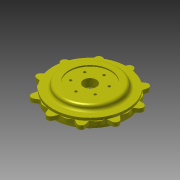
# Autodesk Inventor part: 基准图-主动轮
Saved by Autodesk Inventor 2015 (Build 190159000, 159)
## iProperties
Created: 2017-05-02
Part Number: 基准图-主动轮
Material: 常规
Document SubType Name: Modeling
Designer: Administrator
Density: 1 g/cm^3
Appearance: 黄色
Author: Administrator
Autodesk Inventor part; units mm, degrees
ref_plane "YZ Plane" through (0, 0, 0) normal (1, 0, 0) x (0, 1, 0)
ref_plane "XZ Plane" through (0, 0, 0) normal (0, 1, 0) x (-1, 0, 0)
ref_plane "XY Plane" through (0, 0, 0) normal (0, 0, 1) x (1, 0, 0)
sketch "草图1" plane through (0, 0, 0) normal (0, 0, 1) x (1, 0, 0)
  circle A0 centre (0, 0) radius 141.3842
  line L0 (-50, 166.3842) -> (50, 166.3842)
  line L1 (50, 166.3842) -> (50, 141.3842)
  line L2 (50, 141.3842) -> (-50, 141.3842)
  line L3 (-50, 141.3842) -> (-50, 166.3842)
  line L4 (0, 0) -> (34.0656, 0)
  line L5 (0, 0) -> (0, 40.0691)
  line L6 (-10, 166.3842) -> (-20, 141.3842)
  line L7 (10, 166.3842) -> (20, 141.3842)
  arc A1 (18.8622, 166.3842) -> (13.2913, 158.1558) centre (18.8622, 160.3842) ccw
  arc A2 (18.4913, 145.1558) -> (24.0622, 141.3842) centre (24.0622, 147.3842) ccw
  arc A3 (-13.2913, 158.1558) -> (-18.8622, 166.3842) centre (-18.8622, 160.3842) ccw
  arc A4 (-24.0622, 141.3842) -> (-18.4913, 145.1558) centre (-24.0622, 147.3842) ccw
  circle A5 centre (0, 0) radius 143.3355
  arc A6 (13.2913, 158.1558) -> (-13.2913, 158.1558) centre (0, 152.8393) ccw
  line L8 (-138.249, 105.2184) -> (-57.3473, 163.9969)
  line L9 (-57.3473, 163.9969) -> (-42.6527, 143.7715)
  line L10 (-42.6527, 143.7715) -> (-123.5544, 84.9929)
  line L11 (-123.5544, 84.9929) -> (-138.249, 105.2184)
  line L12 (-173.6916, 3.8627) -> (-142.7899, 98.9684)
  line L13 (-142.7899, 98.9684) -> (-119.0135, 91.2429)
  line L14 (-119.0135, 91.2429) -> (-149.9152, -3.8627)
  line L15 (-149.9152, -3.8627) -> (-173.6916, 3.8627)
  line L16 (-142.7899, -98.9684) -> (-173.6916, -3.8627)
  line L17 (-173.6916, -3.8627) -> (-149.9152, 3.8627)
  line L18 (-149.9152, 3.8627) -> (-119.0135, -91.2429)
  line L19 (-119.0135, -91.2429) -> (-142.7899, -98.9684)
  line L20 (-57.3473, -163.9969) -> (-138.249, -105.2184)
  line L21 (-138.249, -105.2184) -> (-123.5544, -84.9929)
  line L22 (-123.5544, -84.9929) -> (-42.6527, -143.7715)
  line L23 (-42.6527, -143.7715) -> (-57.3473, -163.9969)
  line L24 (50, -166.3842) -> (-50, -166.3842)
  line L25 (-50, -166.3842) -> (-50, -141.3842)
  line L26 (-50, -141.3842) -> (50, -141.3842)
  line L27 (50, -141.3842) -> (50, -166.3842)
  line L28 (-105.8883, 128.7298) -> (-99.2839, 102.6265)
  line L29 (-89.708, 140.4855) -> (-66.9232, 126.1379)
  arc A7 (-70.3607, 128.3025) -> (-63.6368, 128.5256) centre (-67.1635, 133.3797) ccw
  arc A8 (-102.5703, 100.2388) -> (-100.2803, 106.5646) centre (-106.097, 105.0929) ccw
  arc A9 (-82.2087, 135.7632) -> (-103.7146, 120.1383) centre (-89.8367, 123.6496) ccw
  line L30 (-161.3309, 41.905) -> (-140.6447, 24.669)
  line L31 (-155.1506, 60.9261) -> (-128.284, 62.7112)
  arc A10 (-132.3373, 62.4419) -> (-127.0287, 66.5746) centre (-132.7351, 68.4287) ccw
  arc A11 (-141.9, 20.8056) -> (-143.7655, 27.2693) centre (-147.6063, 22.6597) ccw
  arc A12 (-146.3079, 61.5137) -> (-154.5224, 36.232) centre (-145.3588, 47.2299) ccw
  line L32 (-155.1506, -60.9261) -> (-128.284, -62.7112)
  line L33 (-161.3309, -41.905) -> (-140.6447, -24.669)
  arc A13 (-143.7655, -27.2693) -> (-141.9, -20.8056) centre (-147.6063, -22.6597) ccw
  arc A14 (-127.0287, -66.5746) -> (-132.3373, -62.4419) centre (-132.7351, -68.4287) ccw
  arc A15 (-154.5224, -36.232) -> (-146.3079, -61.5137) centre (-145.3588, -47.2299) ccw
  line L34 (-89.708, -140.4855) -> (-66.9232, -126.1379)
  line L35 (-105.8883, -128.7298) -> (-99.2839, -102.6265)
  arc A16 (-100.2803, -106.5646) -> (-102.5703, -100.2388) centre (-106.097, -105.0929) ccw
  arc A17 (-63.6368, -128.5256) -> (-70.3607, -128.3025) centre (-67.1635, -133.3797) ccw
  arc A18 (-103.7146, -120.1383) -> (-82.2087, -135.7632) centre (-89.8367, -123.6496) ccw
  line L36 (10, -166.3842) -> (20, -141.3842)
  line L37 (-10, -166.3842) -> (-20, -141.3842)
  arc A19 (-18.4913, -145.1558) -> (-24.0622, -141.3842) centre (-24.0622, -147.3842) ccw
  arc A20 (24.0622, -141.3842) -> (18.4913, -145.1558) centre (24.0622, -147.3842) ccw
  arc A21 (-13.2913, -158.1558) -> (13.2913, -158.1558) centre (0, -152.8393) ccw
  line L38 (105.8883, -128.7298) -> (99.2839, -102.6265)
  line L39 (89.708, -140.4855) -> (66.9232, -126.1379)
  arc A22 (70.3607, -128.3025) -> (63.6368, -128.5256) centre (67.1635, -133.3797) ccw
  arc A23 (102.5703, -100.2388) -> (100.2803, -106.5646) centre (106.097, -105.0929) ccw
  arc A24 (82.2087, -135.7632) -> (103.7146, -120.1383) centre (89.8367, -123.6496) ccw
  line L40 (161.3309, -41.905) -> (140.6447, -24.669)
  line L41 (155.1506, -60.9261) -> (128.284, -62.7112)
  arc A25 (132.3373, -62.4419) -> (127.0287, -66.5746) centre (132.7351, -68.4287) ccw
  arc A26 (141.9, -20.8056) -> (143.7655, -27.2693) centre (147.6063, -22.6597) ccw
  arc A27 (146.3079, -61.5137) -> (154.5224, -36.232) centre (145.3588, -47.2299) ccw
  line L42 (155.1506, 60.9261) -> (128.284, 62.7112)
  line L43 (161.3309, 41.905) -> (140.6447, 24.669)
  arc A28 (143.7655, 27.2693) -> (141.9, 20.8056) centre (147.6063, 22.6597) ccw
  arc A29 (127.0287, 66.5746) -> (132.3373, 62.4419) centre (132.7351, 68.4287) ccw
  arc A30 (154.5224, 36.232) -> (146.3079, 61.5137) centre (145.3588, 47.2299) ccw
  line L44 (89.708, 140.4855) -> (66.9232, 126.1379)
  line L45 (105.8883, 128.7298) -> (99.2839, 102.6265)
  arc A31 (100.2803, 106.5646) -> (102.5703, 100.2388) centre (106.097, 105.0929) ccw
  arc A32 (63.6368, 128.5256) -> (70.3607, 128.3025) centre (67.1635, 133.3797) ccw
  arc A33 (103.7146, 120.1383) -> (82.2087, 135.7632) centre (89.8367, 123.6496) ccw
  line L46 (57.3473, 163.9969) -> (42.6527, 143.7715)
  line L47 (42.6527, 143.7715) -> (123.5544, 84.9929)
  line L48 (123.5544, 84.9929) -> (138.249, 105.2184)
  line L49 (138.249, 105.2184) -> (57.3473, 163.9969)
  line L50 (23.5706, 141.3842) -> (45.9385, 141.3842)
  line L51 (45.9385, 141.3842) -> (64.0345, 128.2367)
  arc A34 (64.0345, 128.2367) -> (23.5706, 141.3842) centre (0, 0) ccw
  point P0 (0, 166.3842)
  point P1 (0, 141.3842)
  point P2 (-97.7982, 134.6076)
  point P3 (-83.1035, 114.3822)
  point P4 (-105.8883, 128.7298)
  point P5 (-113.058, 123.5207)
  point P6 (-102.5703, 100.2388)
  point P7 (-82.5383, 145.6945)
  point P8 (-63.6368, 128.5256)
  point P9 (-158.2408, 51.4155)
  point P10 (-134.4643, 43.6901)
  point P11 (-161.3309, 41.905)
  point P12 (-155.1506, 60.9261)
  point P13 (-128.284, 62.7112)
  point P14 (-164.0695, 33.4765)
  point P15 (-141.9, 20.8056)
  point P16 (-152.412, 69.3546)
  point P17 (-127.0287, 66.5746)
  point P18 (-158.2408, -51.4155)
  point P19 (-134.4643, -43.6901)
  point P20 (-155.1506, -60.9261)
  point P21 (-128.284, -62.7112)
  point P22 (-161.3309, -41.905)
  point P23 (-140.6447, -24.669)
  point P24 (-152.412, -69.3546)
  point P25 (-127.0287, -66.5746)
  point P26 (-164.0695, -33.4765)
  point P27 (-141.9, -20.8056)
  point P28 (-97.7982, -134.6076)
  point P29 (-83.1035, -114.3822)
  point P30 (-89.708, -140.4855)
  point P31 (-66.9232, -126.1379)
  point P32 (-105.8883, -128.7298)
  point P33 (-99.2839, -102.6265)
  point P34 (-82.5383, -145.6945)
  point P35 (-63.6368, -128.5256)
  point P36 (-113.058, -123.5207)
  point P37 (-102.5703, -100.2388)
  point P38 (0, -166.3842)
  point P39 (0, -141.3842)
  point P40 (10, -166.3842)
  point P41 (20, -141.3842)
  point P42 (-10, -166.3842)
  point P43 (-20, -141.3842)
  point P44 (18.8622, -166.3842)
  point P45 (24.0622, -141.3842)
  point P46 (-18.8622, -166.3842)
  point P47 (-24.0622, -141.3842)
  point P48 (-50, 153.8842)
  point P49 (50, 153.8842)
  dimension "d18" = 286.671
  dimension "d0" = 100
  dimension "d1" = 25
  dimension "d2" = 34.0656
  dimension "d3" = 40.0691
  dimension "d4" = 20
  dimension "d5" = 40
  dimension "d6" = 12
  dimension "d7" = 12
  dimension "d8" = 12
  dimension "d9" = 12
  dimension "d12" = 180
  dimension "d16" = 360
  dimension "d19" = 100
  dimension "d20" = 25
  constraints: 104 end point, 89 point on line, 66 point on circle, 33 centre point, 9 tangent, 6 midpoint, 4 perpendicular, 2 coincident, 2 collinear, 2 horizontal, 2 parallel, 1 equal length, 1 vertical, 1 vertical alignment, 281 other
  measures "d0" distance of L0.start L0.end
  measures "d1" distance of L0.end L1.end
  measures "d2" distance of L4.start L4.end
  measures "d3" distance of L4.start L5.end
  measures "d4" distance of L7.start L6.start
  measures "d5" distance of L7.end L6.end
  measures "d6" diameter of A1
  measures "d7" diameter of A2
  measures "d8" diameter of A3
  measures "d9" diameter of A4
  measures "d19" distance from line of L48 L46.start
  measures "d20" distance from line of L47 L46.start
extrude "拉伸1" add sketch "草图1" against normal blind 15 contours L2 L6 A5 L7 | L7 A5 L2 | L2 A5 L6 | A5 L2 L47 | A5 A2 L2 | A5 L6 A6 L0 L7 | L7 A2 A5 | L2 A4 A5 | A5 A4 L6 | L0 A6
pattern_circular "环形阵列1" count 10 over 360 about axis through (0, 0, -10) along (0, 0, 1) of "拉伸1"
sketch "草图2" plane through (0, 0, 0) normal (0, 0, 1) x (1, 0, 0)
  circle A0 centre (0, 0) radius 143.3355
  arc A1 (64.0345, 128.2367) -> (23.5706, 141.3842) centre (0, 0) ccw projected
  constraints: 1 centre point, 1 coincident, 1 concentric
extrude "拉伸2" add sketch "草图2" against normal blind 15
fillet "圆角1" radius 24 1 edges at (-45.9385, 141.3842, -7.5)
pattern_circular "环形阵列2" count 10 over 360 about axis through (0, 0, -10) along (0, 0, 1) of "圆角1"
sketch "草图3" plane through (0, 0, 0) normal (0, 0, 1) x (1, 0, 0)
  circle A0 centre (0, 0) radius 143.3355
  arc A1 (-70.3607, 128.3025) -> (-63.6368, 128.5256) centre (-67.1635, 133.3797) ccw projected
  constraints: 1 centre point, 1 coincident, 1 tangent
extrude "拉伸3" add sketch "草图3" along normal blind 10
pattern_linear "矩形阵列1" count 2 spacing 25 along (0, 0, -1) of "拉伸3"
sketch "草图4" plane through (0, 0, 10) normal (0, 0, 1) x (1, 0, 0)
  circle A0 centre (0, 0) radius 110
  dimension "d37" = 220
  constraints: 1 centre point, 1 coincident
  measures "d37" diameter of A0
extrude "拉伸4" add sketch "草图4" along normal blind 20
sketch "草图5" plane through (0, 0, -25) normal (0, 0, -1) x (-1, 0, 0)
  circle A0 centre (0, 0) radius 80
  dimension "d40" = 160
  constraints: 1 centre point, 1 coincident
  measures "d40" diameter of A0
extrude "拉伸5" cut sketch "草图5" against normal blind 20
fillet "圆角2" radius 10 4 edges at (80, 0, -25) (80, 0, -5) (-110, 0, 10) (-110, 0, 30)
sketch "草图6" plane through (0, 0, -5) normal (0, 0, -1) x (-1, 0, 0)
  circle A0 centre (0, 55) radius 5
  line L0 (0, 0) -> (0, 9.8996)
  dimension "d44" = 10
  dimension "d45" = 9.8996
  dimension "d46" = 55
  constraints: 2 end point, 1 centre point, 1 point on line, 1 vertical
  measures "d44" diameter of A0
  measures "d45" distance of L0.start L0.end
  measures "d46" distance of L0.start A0.centre
extrude "拉伸6" cut sketch "草图6" against normal through all
pattern_circular "环形阵列3" count 6 over 360 about axis through (0, 0, -10) along (0, 0, 1) of "拉伸6"
sketch "草图7" plane through (0, 0, -5) normal (0, 0, -1) x (-1, 0, 0)
  circle A0 centre (0, 0) radius 25
  dimension "d52" = 50
  constraints: 1 centre point, 1 coincident
  measures "d52" diameter of A0
extrude "拉伸7" cut sketch "草图7" against normal through all
sketch "草图8" plane through (0, 0, 30) normal (0, 0, 1) x (1, 0, 0)
  circle A0 centre (0, 0) radius 80
  dimension "d55" = 160
  constraints: 1 centre point, 1 coincident
  measures "d55" diameter of A0
extrude "拉伸8" cut sketch "草图8" against normal blind 5
equation "\"d53\" = d52"
